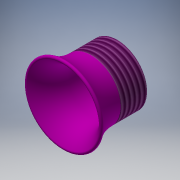
# Autodesk Inventor part: Component 1(Venturi)
Saved by Autodesk Inventor 2018 (Build 220112000, 112)
## iProperties
Created: 2023-03-12
Part Number: Component 1(Venturi)
Material: Generic
Document SubType Name: Modeling
Designer: Habib Mohamed
Density: 1 g/cm^3
Appearance: Magenta
Author: Habib Mohamed
Autodesk Inventor part; units mm, degrees
ref_plane "YZ Plane" through (0, 0, 0) normal (1, 0, 0) x (0, 1, 0)
ref_plane "XZ Plane" through (0, 0, 0) normal (0, 1, 0) x (-1, 0, 0)
ref_plane "XY Plane" through (0, 0, 0) normal (0, 0, 1) x (1, 0, 0)
sketch "Sketch1" plane through (0, 0, 0) normal (1, 0, 0) x (0, 1, 0)
  line L0 (0, 0) -> (0, -10.5356) construction
  line L1 (3.5, -8.28) -> (3.5, -4.28)
  line L2 (3.5, 0) -> (5.87, 0) construction
  line L3 (5.87, 0) -> (5.87, -8.28) construction
  line L4 (4.5, -8.28) -> (3.5, -8.28)
  line L5 (4.5, -4.28) -> (4.5, -8.28)
  line L6 (4.5, -4.28) -> (0, -4.28) construction
  arc A0 (5.8182, -0.4024) -> (5.4586, -0.0591) centre (5.62, -0.25) ccw
  arc A1 (5.4586, -0.0591) -> (3.5, -4.28) centre (9.0275, -4.28) ccw
  arc A2 (5.8182, -0.4024) -> (4.5, -4.28) centre (10.8623, -4.28) ccw
  dimension "d0" = 8.28
  dimension "d1" = 5.87
  dimension "d2" = 3.5
  dimension "d4" = 4.5
  dimension "d5" = 4
  dimension "d6" = 0.5
  dimension "d7" = 6.3623
  constraints: 14 end point, 6 point on circle, 6 tangent, 5 perpendicular, 3 centre point, 3 point on line, 2 vertical
  measures "d0" distance of L1.start L2.start
  measures "d1" distance between parallel lines of L0 L3
  measures "d2" distance between parallel lines of L0 L1
  measures "d4" distance between parallel lines of L0 L5
  measures "d5" distance between parallel lines of L4 L6
  measures "d6" diameter of A0
  measures "d7" radius of A2
revolve "Revolution1" add sketch "Sketch1" angle 360 about axis through (0, 0, 0) along (0, 0, -1)
thread "Thread1" size "M9x0.75" class "6g" standard "ANSI Metric M Profile" full length
body "Solid1"
